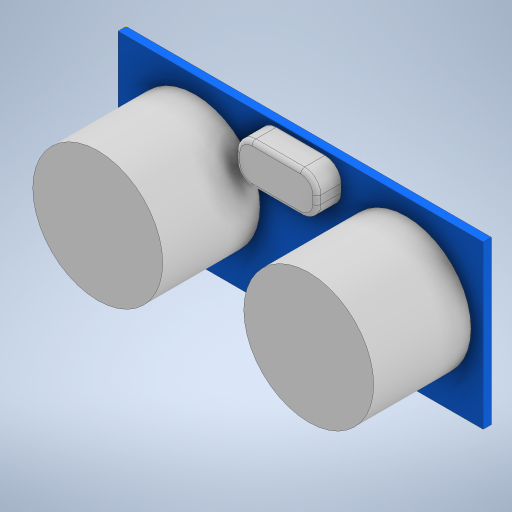
# Autodesk Inventor part: UltrasonicSensor
Saved by Autodesk Inventor 2024.2 (Build 282272000, 272)
## iProperties
Created: 2024-04-02
Part Number: UltrasonicSensor
Material: Generic
Document SubType Name: Modeling
Designer: ringl
Density: 1 g/cm^3
Appearance: Default
Author: ringl
Autodesk Inventor part; units mm, degrees
ref_plane "YZ Plane" through (0, 0, 0) normal (1, 0, 0) x (0, 1, 0)
ref_plane "XZ Plane" through (0, 0, 0) normal (0, 1, 0) x (-1, 0, 0)
ref_plane "XY Plane" through (0, 0, 0) normal (0, 0, 1) x (1, 0, 0)
sketch "Sketch1" plane through (0, 0, 0) normal (0, 0, 1) x (1, 0, 0)
  line L0 (0, 0) -> (45, 0)
  line L1 (45, 0) -> (45, -20)
  line L2 (45, -20) -> (0, -20)
  line L3 (0, -20) -> (0, 0)
  dimension "d0" = 45
  dimension "d1" = 20
  constraints: 8 end point, 2 parallel, 1 horizontal, 1 perpendicular
  measures "d0" distance of L1.end L2.end
  measures "d1" distance of L0.end L1.end
extrude "Extrusion1" add sketch "Sketch1" along normal blind 1
sketch "Sketch2" plane through (0, 0, 1) normal (0, 0, 1) x (1, 0, 0)
  circle A0 centre (9.5, -10) radius 8
  circle A1 centre (35.5, -10) radius 8
  line L0 (0, -20) -> (45, -20) projected
  line L1 (0, 0) -> (0, -20) projected
  dimension "d4" = 16
  dimension "d5" = 16
  dimension "d6" = 26
  dimension "d7" = 10
  dimension "d8" = 9.5
  constraints: 2 centre point, 1 horizontal alignment
  measures "d4" diameter of A0
  measures "d5" diameter of A1
  measures "d6" distance of A1.centre A0.centre
  measures "d7" distance from line of L0 A0.centre
  measures "d8" distance from line of L1 A0.centre
extrude "Extrusion2" add sketch "Sketch2" along normal blind 12
sketch "Sketch3" plane through (0, 0, 1) normal (0, 0, 1) x (1, 0, 0)
  line L0 (17.5, -0.5) -> (27.5, -0.5)
  line L1 (27.5, -0.5) -> (27.5, -5.5)
  line L2 (27.5, -5.5) -> (17.5, -5.5)
  line L3 (17.5, -5.5) -> (17.5, -0.5)
  line L4 (0, 0) -> (0, -20) projected
  line L5 (45, 0) -> (0, 0) projected
  dimension "d11" = 10
  dimension "d12" = 5
  dimension "d13" = 17.5
  dimension "d14" = 0.5
  constraints: 8 end point, 2 parallel, 1 horizontal, 1 perpendicular
  measures "d11" distance of L1.end L2.end
  measures "d12" distance of L0.end L1.end
  measures "d13" distance between parallel lines of L4 L3
  measures "d14" distance between parallel lines of L5 L0
extrude "Extrusion3" add sketch "Sketch3" along normal blind 3
fillet "Fillet1" radius 2 4 edges at (27.5, -0.5, 2.5) (27.5, -5.5, 2.5) (17.5, -0.5, 2.5) (17.5, -5.5, 2.5)
fillet "Fillet2" radius 0.5 8 edges at (17.5, -3, 4) (18.0858, -1.0858, 4) (22.5, -0.5, 4) (26.9142, -1.0858, 4) (27.5, -3, 4) (26.9142, -4.9142, 4) (22.5, -5.5, 4) (18.0858, -4.9142, 4)
sketch "Sketch4" plane through (0, 0, 0) normal (0, 0, -1) x (-1, 0, 0)
  point P0 (0, 0)
body "Solid1"
